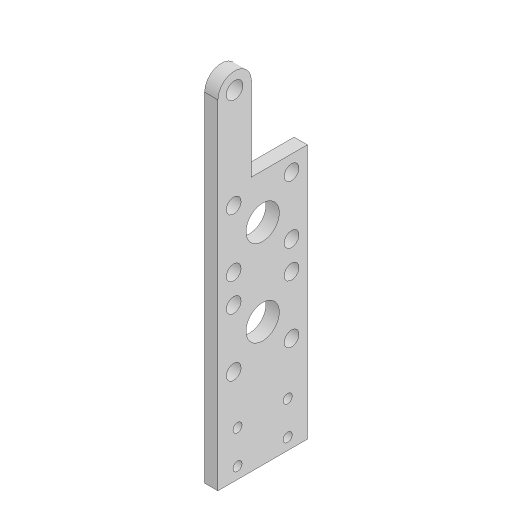
# Autodesk Inventor part: VertialIntakeSlides
Saved by Autodesk Inventor 2023 (Build 270158000, 158)
## iProperties
Created: 2022-11-08
Part Number: VertialIntakeSlides
Material: Generic
Document SubType Name: Modeling
Designer: deli
Density: 1 g/cm^3
Appearance: Default
Author: deli
Autodesk Inventor part; units mm, degrees
ref_plane "YZ Plane" through (0, 0, 0) normal (1, 0, 0) x (0, 1, 0)
ref_plane "XZ Plane" through (0, 0, 0) normal (0, 1, 0) x (-1, 0, 0)
ref_plane "XY Plane" through (0, 0, 0) normal (0, 0, 1) x (1, 0, 0)
sketch "Sketch1" plane through (0, 0, 0) normal (1, 0, 0) x (0, 1, 0)
  line L0 (-49.9062, -175.9546) -> (-110.8778, -175.9546)
  line L1 (-110.8778, -175.9546) -> (-110.8778, -197.3402)
  line L2 (-49.9462, -197.3402) -> (-110.8778, -197.3402)
  circle A0 centre (-100.1278, -180.6474) radius 1.1
  circle A1 centre (-100.1278, -192.6474) radius 1.1
  circle A2 centre (-108.1278, -180.6474) radius 1.1
  circle A3 centre (-108.1278, -192.6474) radius 1.1
  line L3 (-100.1278, -180.6474) -> (-108.1278, -180.6474) construction
  line L4 (-108.1278, -180.6474) -> (-108.1278, -192.6474) construction
  line L5 (-108.1278, -192.6474) -> (-100.1278, -192.6474) construction
  line L6 (-100.1278, -192.6474) -> (-100.1278, -180.6474) construction
  circle A4 centre (-81.213, -186.6474) radius 4
  circle A5 centre (-74.2982, -179.7326) radius 1.778
  circle A6 centre (-74.2982, -193.5622) radius 1.778
  circle A7 centre (-88.1278, -193.5622) radius 1.778
  circle A8 centre (-88.1278, -179.7326) radius 1.778
  line L7 (-74.2982, -179.7326) -> (-88.1278, -193.5622) construction
  line L8 (-74.2982, -193.5622) -> (-88.1278, -179.7326) construction
  line L9 (-88.1278, -179.7326) -> (-88.1278, -193.5622) construction
  line L10 (-74.2982, -179.7326) -> (-74.2982, -193.5622) construction
  circle A9 centre (-67.5538, -179.7326) radius 1.778
  line L11 (-67.5538, -179.7326) -> (-67.5538, -193.5622) construction
  circle A10 centre (-53.7242, -179.7326) radius 1.778
  circle A11 centre (-67.5538, -193.5622) radius 1.778
  circle A12 centre (-60.639, -186.6474) radius 4
  line L12 (-53.7242, -179.7326) -> (-67.5538, -193.5622) construction
  line L13 (-53.7242, -193.5622) -> (-67.5538, -179.7326) construction
  line L14 (-53.7242, -179.7326) -> (-53.7242, -193.5622) construction
  circle A13 centre (-53.7242, -193.5622) radius 1.778
  line L15 (-60.639, -186.6474) -> (-81.213, -186.6474) construction
  line L16 (-49.9462, -183.9546) -> (-49.9462, -197.3402)
  line L17 (-49.9062, -175.9546) -> (-29.9462, -175.9546)
  line L18 (-29.9462, -183.9546) -> (-49.9462, -183.9546)
  arc A14 (-29.9462, -183.9546) -> (-29.9462, -175.9546) centre (-29.9462, -179.9546) ccw
  circle A15 centre (-29.9462, -179.9546) radius 2
  point P0 (0, 0)
  point P1 (-110.8778, -190.5201)
  dimension "d4" = 2.2
  dimension "d5" = 12
  dimension "d6" = 8
  dimension "d7" = 2.75
  dimension "d18" = 8
  dimension "d19" = 3.556
  dimension "d20" = 19.558
  dimension "d21" = 45
  dimension "d22" = 8
  dimension "d23" = 3.556
  dimension "d24" = 19.558
  dimension "d25" = 45
  dimension "d26" = 20.574
  dimension "d27" = 13.8296
  dimension "d28" = 12
  dimension "d29" = 6
  dimension "d30" = 2
  dimension "d31" = 2
  dimension "d32" = 2
  dimension "d33" = 4
  dimension "d34" = 4
  dimension "d35" = 20
  constraints: 38 end point, 16 centre point, 9 equal radius, 7 perpendicular, 5 coincident, 4 equal length, 4 horizontal, 4 midpoint, 2 point on circle, 2 tangent, 2 vertical, 1 parallel, 1 point on line
  measures "d4" diameter of A0
  measures "d5" distance of L5.end L3.start
  measures "d6" distance of L3.start L3.end
  measures "d7" distance between parallel lines of L1 L4
  measures "d18" diameter of A4
  measures "d19" diameter of A5
  measures "d20" distance of L10.start L9.end
  measures "d21" angle of L9 L8
  measures "d22" diameter of A12
  measures "d23" diameter of A10
  measures "d24" distance of L14.start L11.end
  measures "d25" angle of L11 L13
  measures "d26" distance of A12.centre A4.centre
  measures "d27" distance of L14.start L14.end
  measures "d28" horizontal distance of L9.start L3.start
  measures "d29" distance from line of L5 A4.centre
  measures "d30" distance edge to line of A8 L0
  measures "d31" distance edge to line of A7 L2
  measures "d32" distance edge to line of A13 L16
  measures "d33" radius of A14
  measures "d34" diameter of A15
  measures "d35" distance of L18.start L16.start
extrude "Extrusion1" add sketch "Sketch1" along normal blind 3.175
equation "\"d7\" = -0.5 * d6 + 0.5 * d2"
equation "\"d29\" = 0.5 * d5"
equation "\"d2\" = 13.5"
body "Solid1"
